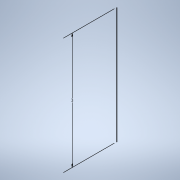
# Autodesk Inventor part: roll
Saved by Autodesk Inventor 2022 (Build 260153000, 153)
## iProperties
Created: 2024-07-28
Part Number: roll
Material: Типовые
Document SubType Name: Modeling
Designer: Капустяник Андрей
Density: 1 g/cm^3
Appearance: По умолчанию
Author: Капустяник Андрей
Autodesk Inventor part; units mm, degrees
ref_plane "YZ Plane" through (0, 0, 0) normal (1, 0, 0) x (0, 1, 0)
ref_plane "XZ Plane" through (0, 0, 0) normal (0, 1, 0) x (-1, 0, 0)
ref_plane "XY Plane" through (0, 0, 0) normal (0, 0, 1) x (1, 0, 0)
sketch "Эскиз1" plane through (0, 0, 0) normal (1, 0, 0) x (0, 1, 0)
  line L0 (0, 0) -> (3, 0)
  line L1 (3, -3.25) -> (3, 3.25)
  line L2 (0, -3.25) -> (0, 3.25)
  line L3 (0, 0) -> (1, 0)
  line L4 (1, 0) -> (1, -3.25)
  line L5 (1, -3.25) -> (0, -3.25)
  line L6 (1, 0) -> (1, 3.25)
  line L7 (1, 3.25) -> (0, 3.25)
  line L8 (1, 0) -> (3, 0)
  line L9 (2, -3) -> (2, 3)
  spline S0 degree 2 poles (3, -3.25) (2, -2.75) (1, -3.25) knots 0 0 0 1 1 1
  spline S1 degree 2 poles (3, 3.25) (2, 2.75) (1, 3.25) knots 0 0 0 1 1 1
  point P0 (2, 0)
  dimension "d0" = 3
  dimension "d1" = 6.5
  dimension "d2" = 6.5
  dimension "d3" = 1
  dimension "d4" = 6
  constraints: 20 end point, 4 midpoint, 3 perpendicular, 3 vertical, 2 point on line, 1 horizontal, 6 other
  measures "d0" distance of L0.end L0.start
  measures "d1" distance of L1.start L1.end
  measures "d2" distance of L2.start L2.end
  measures "d3" distance of L0.start L3.end
  measures "d4" distance of L9.start L9.end
revolve "Вращение1" add sketch "Эскиз1" angle 360 about axis through (0, 1, 0) along (0, 1, 0) contours L2 L7 L6 L0 | L6 S1 L9 L0 | L9 S1 L1 L0
fillet "Сопряжение1" radius 0.3 3 edges at (0, 3, -3.25) (0, 1, -3.25) (0, 0, -3.25)
